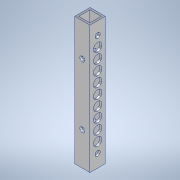
# Autodesk Inventor part: 前後直動12x12_2
Saved by Autodesk Inventor 2020.3 (Build 243373000, 373)
## iProperties
Created: 2020-07-05
Part Number: 前後直動12x12_2
Material: アルミニウム 6061
Document SubType Name: Modeling
Designer: totot
Density: 2.7 g/cm^3
Appearance: アルミニウム - フラット
Mass: 7.39838 g
Surface Area: 47.3226 cm^2
Volume: 2.74014 cm^3
Author: totot
Autodesk Inventor part; units mm, degrees
ref_plane "YZ Plane" through (0, 0, 0) normal (1, 0, 0) x (0, 1, 0)
ref_plane "XZ Plane" through (0, 0, 0) normal (0, 1, 0) x (-1, 0, 0)
ref_plane "XY Plane" through (0, 0, 0) normal (0, 0, 1) x (1, 0, 0)
sketch "スケッチ1" plane through (0, 0, 0) normal (0, 1, 0) x (-1, 0, 0)
  line L0 (0, 0) -> (9, 0)
  line L1 (9, 0) -> (9, -9)
  line L2 (9, -9) -> (0, -9)
  line L3 (0, -9) -> (0, 0)
  line L4 (1.2, -1.2) -> (7.8, -1.2)
  line L5 (7.8, -1.2) -> (7.8, -7.8)
  line L6 (7.8, -7.8) -> (1.2, -7.8)
  line L7 (1.2, -7.8) -> (1.2, -1.2)
  dimension "d0" = 9
  dimension "d1" = 9
  dimension "d2" = 6.6
  dimension "d3" = 6.6
  dimension "d4" = 1.2
  dimension "d5" = 1.2
  constraints: 16 end point, 4 parallel, 2 horizontal, 2 perpendicular
  measures "d0" distance of L1.end L2.end
  measures "d1" distance of L0.end L1.end
  measures "d2" distance of L5.end L6.end
  measures "d3" distance of L6.end L4.start
  measures "d4" distance between parallel lines of L6 L2
  measures "d5" distance between parallel lines of L7 L3
extrude "押し出し1" add sketch "スケッチ1" along normal blind 75
sketch "スケッチ2" plane through (-9, 0, -9) normal (-1, 0, 0) x (0, 0, 1)
  line L0 (0, 0) -> (9, 0) projected
  line L1 (0, 75) -> (9, 75) projected
  line L2 (0, 0) -> (0, 75) projected
  point P0 (4.5, 7.5)
  point P1 (4.5, 67.5)
  dimension "d8" = 7.5
  dimension "d9" = 7.5
  dimension "d10" = 4.5
  dimension "d11" = 4.5
  measures "d8" distance from line of point (4.5, 7.5) L0
  measures "d9" distance from line of L1 point (4.5, 67.5)
  measures "d10" distance from line of point (4.5, 67.5) L2
  measures "d11" distance from line of point (4.5, 7.5) L2
hole "穴1" at (-9, 7.5, -4.5) at (-9, 67.5, -4.5) direction (1, 0, 0) diameter 3 end through all
sketch "スケッチ3" plane through (0, 0, -9) normal (0, 0, -1) x (-1, 0, 0)
  line L0 (9, 0) -> (9, 75) projected
  line L1 (0, 75) -> (9, 75) projected
  line L2 (0, 0) -> (9, 0) projected
  point P0 (4.5, 19.5)
  point P1 (4.5, 55.5)
  dimension "d19" = 4.5
  dimension "d20" = 4.5
  dimension "d21" = 19.5
  dimension "d22" = 19.5
  measures "d19" distance from line of L0 point (4.5, 19.5)
  measures "d20" distance from line of L0 point (4.5, 55.5)
  measures "d21" distance from line of point (4.5, 55.5) L1
  measures "d22" distance from line of point (4.5, 19.5) L2
hole "穴2" at (-4.5, 19.5, -9) at (-4.5, 55.5, -9) direction (0, 0, 1) diameter 3 end through all
sketch "スケッチ4" plane through (-9, 0, -9) normal (-1, 0, 0) x (0, 0, 1)
  circle A0 centre (4.5, 67.5) radius 1.5 projected
  circle A1 centre (4.5, 7.5) radius 1.5 projected
  line L0 (4.5, 67.5) -> (4.5, 7.5)
  point P0 (9, 0)
  point P1 (4.5, 61.5)
  point P2 (4.5, 55.5)
  point P3 (4.5, 49.5)
  point P4 (4.5, 43.5)
  point P5 (4.5, 37.5)
  point P6 (4.5, 31.5)
  point P7 (4.5, 25.5)
  point P8 (4.5, 19.5)
  point P9 (4.5, 13.5)
  dimension "d30" = 60
  dimension "d31" = 6
  dimension "d34" = 6
  constraints: 2 end point, 2 vertical, 1 point on line, 8 other
  measures "d30" distance of L0.end L0.start
  measures "d31" distance of point (4.5, 61.5) L0.start
  measures "d34" distance of point (4.5, 61.5) point (4.5, 55.5)
hole "穴3" at (-9, 61.5, -4.5) at (-9, 55.5, -4.5) at (-9, 49.5, -4.5) at (-9, 43.5, -4.5) at (-9, 37.5, -4.5) at (-9, 31.5, -4.5) at (-9, 25.5, -4.5) at (-9, 19.5, -4.5) at (-9, 13.5, -4.5) direction (1, 0, 0) diameter 5 end through all
equation "\"d1\" = d0"
equation "\"d3\" = d2"
equation "\"d9\" = d8"
equation "\"d10\" = d11"
equation "\"d19\" = d20"
equation "\"d22\" = d21"
equation "\"d31\" = 0.1 * d30"
